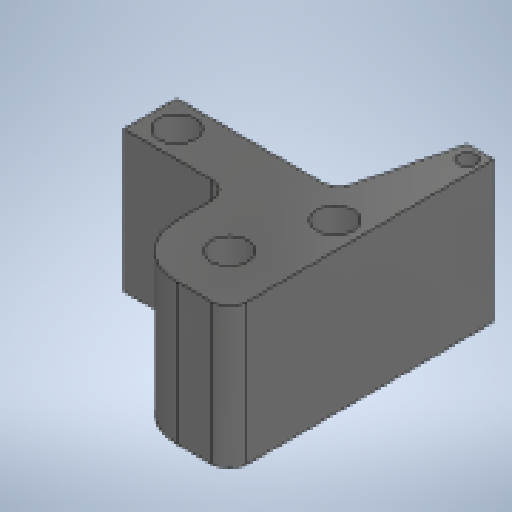
# Autodesk Inventor part: Weapon Link
Saved by Autodesk Inventor 2023.2 (Build 272271000, 271)
## iProperties
Created: 2023-06-29
Part Number: Weapon Link
Material: UHMW, Black
Document SubType Name: Modeling
Designer: Nathan Cai
Density: 0.94 g/cm^3
Appearance: Rubber - Black - Version 1.1
Mass: 18.5873 g
Surface Area: 77.6376 cm^2
Volume: 19.7737 cm^3
Author: Nathan Cai
Autodesk Inventor part; units mm, degrees
ref_plane "YZ Plane" through (0, 0, 0) normal (1, 0, 0) x (0, 1, 0)
ref_plane "XZ Plane" through (0, 0, 0) normal (0, 1, 0) x (-1, 0, 0)
ref_plane "XY Plane" through (0, 0, 0) normal (0, 0, 1) x (1, 0, 0)
sketch "Sketch1" plane through (0, 0, 0) normal (0, 1, 0) x (-1, 0, 0)
  circle A0 centre (0, 0) radius 3.302
  line L0 (-9.525, -9.525) -> (9.525, -9.525)
  line L1 (9.525, -9.525) -> (9.525, 9.525)
  line L2 (9.525, 9.525) -> (-9.525, 9.525)
  line L3 (-9.525, 9.525) -> (-9.525, -9.525)
  line L4 (-9.525, -9.525) -> (9.525, 9.525) construction
  line L5 (9.525, -9.525) -> (-9.525, 9.525) construction
  line L6 (-9.525, -9.525) -> (0, -9.525)
  line L7 (0, -9.525) -> (0, -38.1) construction
  line L8 (0, -38.1) -> (-9.525, -38.1)
  line L9 (-9.525, -38.1) -> (-9.525, -9.525)
  line L10 (-4.7625, -9.525) -> (-4.7625, -38.1) construction
  circle A1 centre (-4.7625, -14.2875) radius 3.302
  line L11 (-9.525, -19.05) -> (0, -19.05)
  line L12 (0, -19.05) -> (0, -9.525)
  line L13 (0, -9.525) -> (-9.525, -9.525)
  line L14 (-9.525, -9.525) -> (-9.525, -19.05)
  line L15 (-9.525, -19.05) -> (0, -9.525) construction
  line L16 (0, -19.05) -> (-9.525, -9.525) construction
  line L17 (-4.7625, -38.1) -> (0, -19.05)
  line L18 (-9.525, -9.525) -> (28.575, -9.525)
  line L19 (28.575, -9.525) -> (28.575, -19.05)
  line L20 (28.575, -19.05) -> (-9.525, -19.05)
  line L21 (-9.525, -19.05) -> (-9.525, -9.525)
  line L22 (-9.525, -14.2875) -> (28.575, -14.2875) construction
  circle A2 centre (23.8125, -14.2875) radius 3.302
  line L23 (-7.1437, -38.1) -> (-7.1438, -19.05) construction
  circle A3 centre (-7.1437, -35.7188) radius 1.5875
  dimension "d0" = 6.604
  dimension "d1" = 19.05
  dimension "d2" = 19.05
  dimension "d3" = 9.525
  dimension "d4" = 47.625
  dimension "d5" = 6.604
  dimension "d6" = 4.7625
  dimension "d7" = 38.1
  dimension "d8" = 6.604
  dimension "d9" = 4.7625
  dimension "d10" = 2.3813
  dimension "d11" = 3.175
  dimension "d12" = 2.3813
  constraints: 48 end point, 8 midpoint, 8 parallel, 6 point on line, 5 perpendicular, 4 centre point, 4 horizontal, 1 coincident
  measures "d0" diameter of A0
  measures "d1" distance of L2.end L1.end
  measures "d2" distance of L1.end L0.end
  measures "d3" distance of L7.end L8.end
  measures "d4" distance between parallel lines of L2 L8
  measures "d5" diameter of A1
  measures "d6" distance from line of L0 A1.centre
  measures "d7" distance of L19.end L20.end
  measures "d8" diameter of A2
  measures "d9" distance from line of L19 A2.centre
  measures "d10" distance between parallel lines of L9 L23
  measures "d11" diameter of A3
  measures "d12" distance from line of L8 A3.centre
extrude "Extrusion1" add sketch "Sketch1" along normal blind 25.4 contours L3 L2 L1 L0 | L0 L12 L11 L9 | L0 L18 L19 L20 L12
fillet "Fillet1" radius 9.525 1 edges at (-9.525, 12.7, 9.525)
fillet "Fillet2" radius 3.175 2 edges at (9.525, 12.7, 9.525) (-9.525, 12.7, -9.525)
equation "\"d10\" = 0.25 * d3"
equation "\"d12\" = d10"
body "Solid1"
